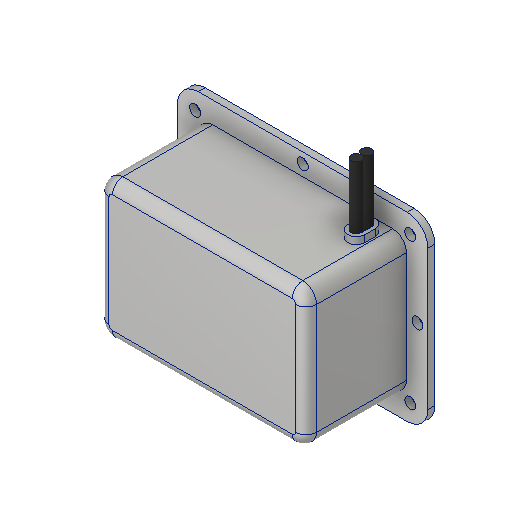
# Autodesk Inventor part: CNCM_ALU_Vibration_module_cover
Saved by Autodesk Inventor 2025 (Build 290162010, 162A)
## iProperties
Created: 2018-09-15
Part Number: CNCM_ALU_Vibration_module_cover
Material: Aluminum 6061
Document SubType Name: Modeling
Designer: Andrzej
Density: 2.7 g/cm^3
Appearance: Aluminum - Flat
Mass: 8.61647 g
Surface Area: 46.3348 cm^2
Volume: 3.19129 cm^3
Author: Andrzej
Autodesk Inventor part; units mm, degrees
ref_plane "YZ Plane" through (0, 0, 0) normal (1, 0, 0) x (0, 1, 0)
ref_plane "XZ Plane" through (0, 0, 0) normal (0, 1, 0) x (-1, 0, 0)
ref_plane "XY Plane" through (0, 0, 0) normal (0, 0, 1) x (1, 0, 0)
sketch "Sketch1" plane through (0, 0, 0) normal (0, 0, 1) x (1, 0, 0)
  line L0 (-15, 10) -> (15, 10)
  line L1 (15, 10) -> (15, -10)
  line L2 (15, -10) -> (-15, -10)
  line L3 (-15, -10) -> (-15, 10)
  line L4 (-18.1, 13.1) -> (18.1, 13.1)
  line L5 (18.1, 13.1) -> (18.1, -13.1)
  line L6 (18.1, -13.1) -> (-18.1, -13.1)
  line L7 (-18.1, -13.1) -> (-18.1, 13.1)
  line L8 (16.6, 11.6) -> (-16.6, 11.6)
  line L9 (-16.6, 11.6) -> (-16.6, -11.6)
  line L10 (-16.6, -11.6) -> (16.6, -11.6)
  line L11 (16.6, -11.6) -> (16.6, 11.6)
  line L12 (13.5, 8.5) -> (-13.5, 8.5)
  line L13 (-13.5, 8.5) -> (-13.5, -8.5)
  line L14 (-13.5, -8.5) -> (13.5, -8.5)
  line L15 (13.5, -8.5) -> (13.5, 8.5)
  point P0 (0, 0)
  dimension "d0" = 20
  dimension "d1" = 30
  dimension "d2" = 3.1
  dimension "d3" = 1.6
  dimension "d4" = 1.5
  dimension "d17" = 15
  dimension "d18" = 10
  constraints: 32 end point, 8 parallel, 4 perpendicular, 1 horizontal, 9 other
  measures "d0" distance of L2.end L0.start
  measures "d1" distance of L1.end L2.end
  measures "d2" distance between parallel lines of L3 L7
  measures "d3" distance between parallel lines of L0 L8
  measures "d4" distance between parallel lines of L0 L12
  measures "d17" distance from line of point (0, 0) L1
  measures "d18" distance from line of point (0, 0) L0
extrude "Extrusion1" add sketch "Sketch1" along normal blind 1 contours L4 L5 L6 L7 | L11 L10 L9 L8
extrude "Extrusion3" add sketch "Sketch1" along normal blind 14 contours L0 L1 L2 L3
sketch "Sketch2" plane through (0, 0, 14) normal (0, 0, 1) x (1, 0, 0)
  line L0 (13.5, 8.5) -> (13.5, -8.5) projected
  line L1 (13.5, -8.5) -> (-13.5, -8.5) projected
  line L2 (-13.5, -8.5) -> (-13.5, 8.5) projected
  line L3 (-13.5, 8.5) -> (13.5, 8.5) projected
  line L4 (15, 10) -> (-15, 10) projected
  line L5 (-15, 10) -> (-15, -10) projected
  line L6 (-15, -10) -> (15, -10) projected
  line L7 (15, -10) -> (15, 10) projected
  point P0 (0, 0)
extrude "Extrusion4" add sketch "Sketch2" along normal blind 1.5 contours L0 L1 L2 L3 | L7 L6 L5 L4
fillet "Fillet1" radius 2 8 edges at (-15, 10, 8.25) (-15, -10, 8.25) (15, 10, 8.25) (15, -10, 8.25) (13.5, -8.5, 7) (-13.5, -8.5, 7) (13.5, 8.5, 7) (-13.5, 8.5, 7)
fillet "Fillet1" radius 3 4 edges at (-18.1, -13.1, 0.5) (18.1, -13.1, 0.5) (18.1, 13.1, 0.5) (-18.1, 13.1, 0.5)
fillet "Fillet2" radius 1.5 8 edges at (-14.4142, 9.4142, 15.5) (-15, 0, 15.5) (-14.4142, -9.4142, 15.5) (0, -10, 15.5) (14.4142, -9.4142, 15.5) (15, 0, 15.5) (14.4142, 9.4142, 15.5) (0, 10, 15.5)
sketch "Sketch3" plane through (0, 0, 1) normal (0, 0, 1) x (1, 0, 0)
  arc A0 (-15.1, 13.1) -> (-18.1, 10.1) centre (-15.1, 10.1) ccw projected
  line L0 (-18.1, 10.1) -> (-18.1, -10.1) projected
  arc A1 (-18.1, -10.1) -> (-15.1, -13.1) centre (-15.1, -10.1) ccw projected
  line L1 (-15.1, -13.1) -> (15.1, -13.1) projected
  arc A2 (15.1, -13.1) -> (18.1, -10.1) centre (15.1, -10.1) ccw projected
  line L2 (18.1, -10.1) -> (18.1, 10.1) projected
  arc A3 (18.1, 10.1) -> (15.1, 13.1) centre (15.1, 10.1) ccw projected
  line L3 (15.1, 13.1) -> (-15.1, 13.1) projected
  line L4 (15, 8) -> (15, -8) projected
  arc A4 (13, -10) -> (15, -8) centre (13, -8) ccw projected
  line L5 (13, -10) -> (-13, -10) projected
  arc A5 (-15, -8) -> (-13, -10) centre (-13, -8) ccw projected
  line L6 (-15, -8) -> (-15, 8) projected
  arc A6 (-13, 10) -> (-15, 8) centre (-13, 8) ccw projected
  line L7 (-13, 10) -> (13, 10) projected
  arc A7 (15, 8) -> (13, 10) centre (13, 8) ccw projected
  line L8 (16.6, -8) -> (16.6, 8)
  arc A8 (16.6, 8) -> (13, 11.6) centre (13, 8) ccw
  line L9 (13, 11.6) -> (-13, 11.6)
  arc A9 (-13, 11.6) -> (-16.6, 8) centre (-13, 8) ccw
  line L10 (-16.6, 8) -> (-16.6, -8)
  arc A10 (-16.6, -8) -> (-13, -11.6) centre (-13, -8) ccw
  line L11 (-13, -11.6) -> (13, -11.6)
  arc A11 (13, -11.6) -> (16.6, -8) centre (13, -8) ccw
  point P0 (0, 0)
  point P1 (15.5456, -10.5456)
  point P2 (0, -11.6)
  point P3 (-15.5456, -10.5456)
  point P4 (-16.6, 0)
  point P5 (16.6, 0)
  point P6 (15.5456, 10.5456)
  point P7 (0, 11.6)
  point P8 (-15.5456, 10.5456)
  dimension "d16" = 1.6
  constraints: 12 point on circle, 8 end point, 4 centre point, 4 midpoint, 7 other
  measures "d16" radial gap between concentric circles of A4 A11
hole "Hole1" at (15.5456, -10.5456, 1) at (0, -11.6, 1) at (-15.5456, -10.5456, 1) at (-16.6, 0, 1) at (16.6, 0, 1) at (15.5456, 10.5456, 1) at (0, 11.6, 1) at (-15.5456, 10.5456, 1) direction (0, 0, -1) diameter 1.6 end through all both
sketch "Sketch4" plane through (-13, 10, 1) normal (0, 1, 0) x (1, 0, 0)
  line L0 (26, -13) -> (0, -13) projected
  line L1 (26, 0) -> (26, -13) projected
  line L2 (0, 0) -> (26, 0) projected
  line L3 (0, -13) -> (0, 0) projected
  line L4 (24.5, -3.75) -> (24.5, -2.25) construction
  line L5 (25.25, -3.75) -> (25.25, -2.25)
  line L6 (23.75, -2.25) -> (23.75, -3.75)
  arc A0 (23.75, -3.75) -> (25.25, -3.75) centre (24.5, -3.75) ccw
  arc A1 (25.25, -2.25) -> (23.75, -2.25) centre (24.5, -2.25) ccw
  line L7 (25.75, -3.75) -> (25.75, -2.25)
  arc A2 (25.75, -2.25) -> (23.25, -2.25) centre (24.5, -2.25) ccw
  line L8 (23.25, -2.25) -> (23.25, -3.75)
  arc A3 (23.25, -3.75) -> (25.75, -3.75) centre (24.5, -3.75) ccw
  circle A4 centre (24.5, -3.75) radius 0.75
  circle A5 centre (24.5, -2.25) radius 0.75
  point P0 (13, 1)
  point P1 (24.5, -3)
  dimension "d26" = 1.5
  dimension "d27" = 1.5
  dimension "d28" = 1.5
  dimension "d29" = 10
  dimension "d30" = 13
  dimension "d31" = 0.5
  constraints: 12 end point, 8 point on circle, 4 centre point, 4 tangent, 2 coincident, 2 horizontal alignment, 2 parallel, 1 midpoint, 1 vertical, 7 other
  measures "d26" distance of L4.start L4.end
  measures "d27" diameter of A1
  measures "d28" distance from line of L1 point (24.5, -3)
  measures "d29" distance from line of L0 point (24.5, -3)
  measures "d30" distance between parallel lines of L0 L2
  measures "d31" radial gap between concentric circles of A0 A3
extrude "Extrusion5" add sketch "Sketch4" along normal blind 1 contours A3 L8 A2 L7
extrude "Extrusion6" add sketch "Sketch4" along normal blind 10 contours A0 A4 | A5 A1
body "Solid1"
